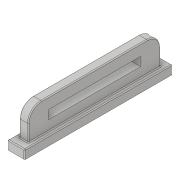
# Autodesk Inventor part: Base
Saved by Autodesk Inventor 2017 (Build 210142000, 142)
## iProperties
Created: 2016-07-28
Part Number: Base
Material: Generic
Document SubType Name: Modeling
Designer: Tutorial Books
Density: 1 g/cm^3
Appearance: Default
Author: Tutorial Books
Autodesk Inventor part; units mm, degrees
ref_plane "YZ Plane" through (0, 0, 0) normal (1, 0, 0) x (0, 1, 0)
ref_plane "XZ Plane" through (0, 0, 0) normal (0, 1, 0) x (-1, 0, 0)
ref_plane "XY Plane" through (0, 0, 0) normal (0, 0, 1) x (1, 0, 0)
sketch "Sketch1" plane through (0, 0, 0) normal (1, 0, 0) x (0, 1, 0)
  line L0 (0, 76.2) -> (19.05, 76.2)
  line L1 (34.29, 60.96) -> (34.29, -60.96)
  line L2 (19.05, -76.2) -> (0, -76.2)
  line L3 (0, -76.2) -> (0, 76.2)
  line L4 (21.59, 53.34) -> (11.43, 53.34)
  line L5 (11.43, 53.34) -> (11.43, -53.34)
  line L6 (11.43, -53.34) -> (21.59, -53.34)
  line L7 (21.59, -53.34) -> (21.59, 53.34)
  line L8 (21.59, 53.34) -> (11.43, -53.34) construction
  line L9 (11.43, 53.34) -> (21.59, -53.34) construction
  arc A0 (34.29, 60.96) -> (19.05, 76.2) centre (19.05, 60.96) ccw
  arc A1 (19.05, -76.2) -> (34.29, -60.96) centre (19.05, -60.96) ccw
  line L10 (0, 0) -> (84.7989, 0) construction
  point P0 (16.51, 0)
  dimension "d0" = 15.24
  dimension "d1" = 152.4
  dimension "d2" = 106.68
  dimension "d3" = 34.29
  dimension "d4" = 11.43
  dimension "d5" = 10.16
  constraints: 22 end point, 4 perpendicular, 4 point on circle, 4 tangent, 3 horizontal, 3 midpoint, 2 centre point, 2 parallel, 1 equal radius, 2 other
  measures "d0" radius of A0
  measures "d1" distance of L2.end L0.start
  measures "d2" distance of L6.end L4.start
  measures "d3" distance between parallel lines of L3 L1
  measures "d4" distance between parallel lines of L3 L5
  measures "d5" distance of L4.start L4.end
extrude "Extrusion1" add sketch "Sketch1" along normal mid plane 10.16
sketch "Sketch3" plane through (0, 0, 0) normal (0, 1, 0) x (-1, 0, 0)
  line L0 (9.906, 85.09) -> (-9.906, 85.09)
  line L1 (-9.906, 85.09) -> (-9.906, -85.09)
  line L2 (-9.906, -85.09) -> (9.906, -85.09)
  line L3 (9.906, -85.09) -> (9.906, 85.09)
  line L4 (9.906, 85.09) -> (-9.906, -85.09) construction
  line L5 (-9.906, 85.09) -> (9.906, -85.09) construction
  point P0 (0, 0)
  dimension "d8" = 170.18
  dimension "d9" = 19.812
  constraints: 12 end point, 2 midpoint, 2 parallel, 1 horizontal, 1 perpendicular
  measures "d8" distance of L0.end L1.end
  measures "d9" distance of L1.end L2.end
extrude "Extrusion2" add sketch "Sketch3" against normal blind 10.16
fillet "Fillet1" radius 1.016 22 edges at (5.08, 29.8263, 71.7363) (5.08, 9.525, 76.2) (5.08, 29.8263, -71.7363) (5.08, 9.525, -76.2) (5.08, 34.29, 0) (-5.08, 34.29, 0) (-5.08, 29.8263, -71.7363) (-5.08, 9.525, -76.2) (-5.08, 9.525, 76.2) (-5.08, 29.8263, 71.7363) (0, 0, 76.2) (5.08, 0, 0) (0, 0, -76.2) (-5.08, 0, 0) (0, 0, 85.09) (9.906, 0, 0) (-9.906, 0, 0) (9.906, -5.08, 85.09) (-9.906, -5.08, 85.09) (9.906, -5.08, -85.09) (0, 0, -85.09) (-9.906, -5.08, -85.09)
body "Solid1"
